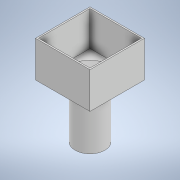
# Autodesk Inventor part: PMT housing
Saved by Autodesk Inventor 2022 (Build 260153000, 153)
## iProperties
Created: 2021-09-24
Part Number: PMT housing
Material: Generic
Document SubType Name: Modeling
Designer: The Shack
Density: 1 g/cm^3
Appearance: Default
Author: The Shack
Autodesk Inventor part; units mm, degrees
ref_plane "YZ Plane" through (0, 0, 0) normal (1, 0, 0) x (0, 1, 0)
ref_plane "XZ Plane" through (0, 0, 0) normal (0, 1, 0) x (-1, 0, 0)
ref_plane "XY Plane" through (0, 0, 0) normal (0, 0, 1) x (1, 0, 0)
sketch "Sketch1" plane through (0, 0, 0) normal (0, 1, 0) x (-1, 0, 0)
  line L0 (-51.9938, 0) -> (-51.9938, 51.9938)
  line L1 (-51.9938, 51.9938) -> (0, 51.9938)
  line L2 (51.9938, 0) -> (51.9938, -51.9938)
  line L3 (51.9938, -51.9938) -> (0, -51.9938)
  line L4 (-51.9938, 0) -> (-51.9938, 51.9938)
  line L5 (-51.9938, 51.9938) -> (0, 51.9938)
  line L6 (-51.9938, 0) -> (-51.9938, -51.9938)
  line L7 (-51.9938, -51.9938) -> (0, -51.9938)
  line L8 (51.9938, 0) -> (51.9938, 51.9938)
  line L9 (51.9938, 51.9938) -> (0, 51.9938)
  point P0 (0, 0)
  dimension "d0" = 51.9938
  dimension "d1" = 51.9938
  dimension "d2" = 51.9938
  dimension "d3" = 51.9938
  dimension "d4" = 51.9938
  dimension "d5" = 51.9938
  dimension "d6" = 51.9938
  dimension "d7" = 51.9938
  dimension "d8" = 51.9938
  dimension "d9" = 51.9938
  constraints: 20 end point
  measures "d0" distance of L0.end L1.end
  measures "d1" distance of L0.start L0.end
  measures "d2" distance of L2.end L3.end
  measures "d3" distance of L2.start L2.end
  measures "d4" distance of L0.end L5.end
  measures "d5" distance of L4.start L0.end
  measures "d6" distance of L7.end L6.end
  measures "d7" distance of L6.end L6.start
  measures "d8" distance of L9.end L8.end
  measures "d9" distance of L8.end L8.start
extrude "Extrusion1" add sketch "Sketch1" against normal blind 3
sketch "Sketch2" plane through (0, 0, 0) normal (0, 1, 0) x (1, 0, 0)
  line L0 (54.991, 0) -> (54.991, -54.991)
  line L1 (54.991, -54.991) -> (0, -54.991)
  line L2 (-54.991, 0) -> (-54.991, -54.991)
  line L3 (-54.991, -54.991) -> (0, -54.991)
  line L4 (-54.991, 0) -> (-54.991, 54.991)
  line L5 (-54.991, 54.991) -> (0, 54.991)
  line L6 (54.991, 0) -> (54.991, 54.991)
  line L7 (54.991, 54.991) -> (0, 54.991)
  line L8 (-51.9938, 51.9938) -> (51.9938, 51.9938) projected
  line L9 (51.9938, 0) -> (51.9938, 51.9938)
  line L10 (51.9938, 51.9938) -> (0, 51.9938)
  line L11 (51.9938, 0) -> (51.9938, -51.9938)
  line L12 (51.9938, -51.9938) -> (0, -51.9938)
  line L13 (-51.9938, 0) -> (-51.9938, -51.9938)
  line L14 (-51.9938, -51.9938) -> (0, -51.9938)
  line L15 (-51.9938, 0) -> (-51.9938, 51.9938)
  line L16 (-51.9938, 51.9938) -> (0, 51.9938)
  point P0 (0, 0)
  dimension "d14" = 54.991
  dimension "d15" = 54.991
  dimension "d16" = 54.991
  dimension "d17" = 54.991
  dimension "d18" = 54.991
  dimension "d19" = 54.991
  dimension "d20" = 51.9938
  dimension "d21" = 51.9938
  dimension "d22" = 51.9938
  dimension "d23" = 51.9938
  dimension "d24" = 51.9938
  dimension "d25" = 51.9938
  dimension "d26" = 51.9938
  dimension "d27" = 51.9938
  constraints: 32 end point, 1 point on line
  measures "d14" distance of L0.end L1.end
  measures "d15" distance of L0.start L0.end
  measures "d16" distance of L3.end L2.end
  measures "d17" distance of L2.end L2.start
  measures "d18" distance of L4.end L5.end
  measures "d19" distance of L4.start L4.end
  measures "d20" distance of L10.end L8.end
  measures "d21" distance of L8.end L9.start
  measures "d22" distance of L11.end L12.end
  measures "d23" distance of L11.start L11.end
  measures "d24" distance of L14.end L13.end
  measures "d25" distance of L13.end L13.start
  measures "d26" distance of L8.start L16.end
  measures "d27" distance of L15.start L8.start
extrude "Extrusion2" add sketch "Sketch2" along normal blind 70 and the other way blind 3
sketch "Sketch3" plane through (0, -3, 0) normal (0, -1, 0) x (1, 0, 0)
  circle A0 centre (0, 0) radius 50.4952
  dimension "d32" = 100.9904
  constraints: 1 centre point, 1 coincident
  measures "d32" diameter of A0
extrude "Extrusion3" add sketch "Sketch3" along normal blind 18
sketch "Sketch4" plane through (0, -21, 0) normal (0, -1, 0) x (1, 0, 0)
  circle A0 centre (0, 0) radius 30
  dimension "d35" = 60
  constraints: 1 centre point, 1 coincident
  measures "d35" diameter of A0
extrude "Extrusion4" add sketch "Sketch4" along normal blind 90
sketch "Sketch6" plane through (0, -111, 0) normal (0, -1, 0) x (1, 0, 0)
  circle A0 centre (0, 0) radius 27.4955
  dimension "d39" = 54.991
  constraints: 1 centre point, 1 coincident
  measures "d39" diameter of A0
hole "Hole1" at (0, -111, 0) direction (0, 1, 0) diameter 54.991 depth 111
chamfer "Chamfer1" distance 20.49 distance2 18 1 edges at (-50.4952, -21, 0) measured on face at (-21.4731, -21, -37.7754)
chamfer "Chamfer2" distance 17 distance2 18 1 edges at (0, 0, 27.4955) measured on face at (-43.7609, 0, -1.1047)
body "Solid1"
